Autodesk Inventor part; units mm, degrees
(part 2 of 2)
  point P135 (-2.7232, -8.3812)
  point P136 (-2.3444, -8.4949)
  point P137 (-1.961, -8.5916)
  point P138 (-1.5735, -8.6709)
  point P139 (-1.1829, -8.7327)
  point P140 (-0.7899, -8.777)
  point P141 (-0.3954, -8.8036)
  point P142 (-4.8548, 7.3547)
  point P143 (-5.1799, 7.1295)
  point P144 (-5.4945, 6.8899)
  point P145 (-5.7981, 6.6364)
  point P146 (-6.09, 6.3696)
  point P147 (-6.3696, 6.09)
  point P148 (-6.6364, 5.7981)
  point P149 (-6.8899, 5.4945)
  point P150 (-7.1295, 5.1799)
  point P151 (-7.3547, 4.8548)
  point P152 (-7.5651, 4.5199)
  point P153 (-7.7602, 4.176)
  point P154 (-7.9398, 3.8236)
  point P155 (-8.1033, 3.4635)
  point P156 (-8.2506, 3.0965)
  point P157 (-8.3812, 2.7232)
  point P158 (-8.4949, 2.3444)
  point P159 (-8.5916, 1.961)
  point P160 (-8.6709, 1.5735)
  point P161 (-8.7327, 1.1829)
  point P162 (-8.777, 0.7899)
  point P163 (-8.8036, 0.3954)
  point P164 (-7.3547, 4.8548)
  point P165 (-7.5651, 4.5199)
  point P166 (-7.7602, 4.176)
  point P167 (-7.9398, 3.8236)
  point P168 (-8.1033, 3.4635)
  point P169 (-8.2506, 3.0965)
  point P170 (-8.3812, 2.7232)
  point P171 (-8.4949, 2.3444)
  point P172 (-8.5916, 1.961)
  point P173 (-8.6709, 1.5735)
  point P174 (-8.7327, 1.1829)
  point P175 (-8.777, 0.7899)
  point P176 (-8.8036, 0.3954)
  point P177 (-8.8125, 0)
  point P178 (-8.8036, -0.3954)
  point P179 (-8.777, -0.7899)
  point P180 (-8.7327, -1.1829)
  point P181 (-8.6709, -1.5735)
  point P182 (-8.5916, -1.961)
  point P183 (-8.4949, -2.3444)
  point P184 (-8.3812, -2.7232)
  point P185 (-8.2506, -3.0965)
  point P186 (-8.1033, -3.4635)
  point P187 (-7.9398, -3.8236)
  point P188 (-7.7602, -4.176)
  point P189 (-7.5651, -4.5199)
  point P190 (-7.3547, -4.8548)
  dimension "d0" = 18
  dimension "d1" = 0.2
  dimension "d2" = 0.2
  dimension "d3" = 0.1
  dimension "d4" = 0.05
  dimension "d5" = 17.625
  dimension "d6" = 12.5
  dimension "d7" = 18
  constraints: 964 point on circle, 772 end point, 388 centre point, 193 coincident, 1 vertical
  measures "d0" diameter of A220
  measures "d1" distance of L221.start L221.end
  measures "d2" distance of L222.start L222.end
  measures "d3" distance of L222.start L221.end
  measures "d4" distance from line of L223 L221.end
  measures "d5" diameter of A221
  measures "d6" diameter of A386
  measures "d7" diameter of A387
extrude "押し出し1" add sketch "スケッチ1" along normal blind 1.5 contours L0 A1 L1 A387 L134 A135 L135 L132 A133 L133 L130 A131 L131 L128 A129 L129 L126 A127 L127 L124 A125 L125 L122 A123 L123 L120 A121 L121 L118 A119 L119 L116 A117 L117 L114 A115 L115 L112 A113 L113 L110 A111 L111 L108 A109 L109 L106 A107 L107 L104 A105 L105 L102 A103 L103 L100 A101 L101 L98 A99 L99 L96 A97 L97 L94 A95 L95 L92 A93 L93 L90 A91 L91 L88 A89 L89 L86 A87 L87 L84 A85 L85 L82 A83 L83 L80 A81 L81 L78 A79 L79 L190 A190 L191 L188 A188 L189 L186 A186 L187 L184 A184 L185 L182 A182 L183 L180 A180 L181 L178 A178 L179 L176 A176 L177 L174 A174 L175 L172 A172 L173 L170 A170 L171 L168 A168 L169 L166 A166 L167 L164 A164 L165 L162 A162 L163 L160 A160 L161 L158 A158 L159 L156 A156 L157 L228 A227 L229 L226 A225 L227 L224 A223 L225 L221 A221 L222 L285 A285 L286 L283 A283 L284 L281 A281 L282 L279 A279 L280 L277 A277 L278 L275 A275 L276 L273 A273 L274 L271 A271 L272 L269 A269 L270 L267 A267 L268 L265 A265 L266 L263 A263 L264 L261 A261 L262 L259 A259 L260 L257 A257 L258 L255 A255 L256 L253 A253 L254 L251 A251 L252 L249 A249 L250 L247 A247 L248 L245 A245 L246 L243 A243 L244 L241 A241 L242 L239 A239 L240 L237 A237 L238 L236 A235 L376 L373 A374 L374 L371 A372 L372 L369 A370 L370 L367 A368 L368 L365 A366 L366 L363 A364 L364 L361 A362 L362 L359 A360 L360 L357 A358 L358 L355 A329 L329 L327 A327 L328 L325 A325 L326 L323 A323 L324 L321 A321 L322 L319 A319 L320 L317 A317 L318 L315 A315 L316 L313 A313 L314 L311 A311 L312 L309 A309 L310 L307 A307 L308 L305 A305 L306 L303 A303 L304 L301 A301 L302 L76 A77 L77 L74 A75 L75 L72 A73 L73 L70 A71 L71 L68 A69 L69 L66 A67 L67 L64 A65 L65 L62 A63 L63 L60 A61 L61 L58 A59 L59 L56 A57 L57 L54 A55 L55 L52 A53 L53 L50 A51 L51 L48 A49 L49 L46 A47 L47 L44 A45 L45 L42 A43 L43 L40 A41 L41 L38 A39 L39 L36 A37 L37 L34 A35 L35 L32 A33 L33 L30 A31 L31 L28 A29 L29 L26 A27 L27 L24 A25 L25 L22 A23 L23 L20 A21 L21 L18 A19 L19 L16 A17 L17 L14 A15 L15 L12 A13 L13 L10 A11 L11 L8 A9 L9 L6 A7 L7 L4 A5 L5 L2 A3 L3
sketch "スケッチ2" plane through (0, 1.5, 0) normal (0, 1, 0) x (1, 0, 0)
  circle A0 centre (0, 0) radius 7.75
  circle A1 centre (0, 0) radius 6.25
  dimension "d10" = 15.5
  dimension "d11" = 12.5
  constraints: 2 centre point, 2 coincident
  measures "d10" diameter of A0
  measures "d11" diameter of A1
extrude "押し出し2" add sketch "スケッチ2" along normal blind 2.6
equation "\"d2\" = d1"
